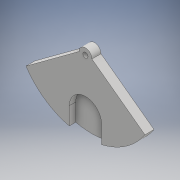
# Autodesk Inventor part: RescueKitThrow-Joint
Saved by Autodesk Inventor 2018.3 (Build 223284000, 284)
## iProperties
Created: 2019-02-13
Part Number: RescueKitThrow-Joint
Material: 一般
Document SubType Name: Modeling
Designer: TOMOKI
Density: 1 g/cm^3
Appearance: 既定
Author: TOMOKI
Autodesk Inventor part; units mm, degrees
ref_plane "YZ Plane" through (0, 0, 0) normal (1, 0, 0) x (0, 1, 0)
ref_plane "XZ Plane" through (0, 0, 0) normal (0, 1, 0) x (-1, 0, 0)
ref_plane "XY Plane" through (0, 0, 0) normal (0, 0, 1) x (1, 0, 0)
sketch "スケッチ1" plane through (0, 0, 0) normal (0, 1, 0) x (-1, 0, 0)
  arc A0 (9.0513, 24.7723) -> (100.9487, 24.7723) centre (55, 55) ccw
  circle A1 centre (55, 15) radius 12.5
  arc A2 (60, 55) -> (50, 55) centre (55, 55) ccw
  circle A3 centre (55, 55) radius 2
  arc A4 (9.0513, 24.7723) -> (100.9487, 24.7723) centre (55, 55) ccw
  line L0 (100.9487, 24.7723) -> (60, 55)
  line L1 (50, 55) -> (9.0513, 24.7723)
  circle A5 centre (55, 55) radius 5
  arc A6 (60, 55) -> (50, 55) centre (55, 55) ccw
  point P0 (0, 0)
  constraints: 8 point on circle, 7 centre point, 4 end point, 3 concentric, 1 coincident
extrude "押し出し1" add sketch "スケッチ1" along normal blind 7
sketch "スケッチ2" plane through (0, 7, 0) normal (0, 1, 0) x (1, 0, 0)
  circle A0 centre (-55, -15) radius 12.5 projected
  circle A1 centre (-55, -15) radius 12.5
  point P0 (0, 0)
  constraints: 1 centre point, 1 coincident
extrude "押し出し2" add sketch "スケッチ2" against normal blind 2
sketch "スケッチ3" plane through (0, 0, 0) normal (0, -1, 0) x (1, 0, 0)
  circle A0 centre (-55, 15) radius 12.5 projected
  line L0 (-67.5, 15) -> (-42.5, 15)
  line L1 (-42.5, 15) -> (-42.5, -1.7653)
  line L2 (-42.5, -1.7653) -> (-67.5, -1.7653)
  line L3 (-67.5, -1.7653) -> (-67.5, 15)
  point P0 (0, 0)
  constraints: 8 end point, 2 parallel, 1 horizontal, 1 horizontal alignment, 1 perpendicular, 1 other
extrude "押し出し3" cut sketch "スケッチ3" against normal blind 5 contours L1 L2 L3 A0 | A0 L0 picked at (-57.3669, 11.5709)
